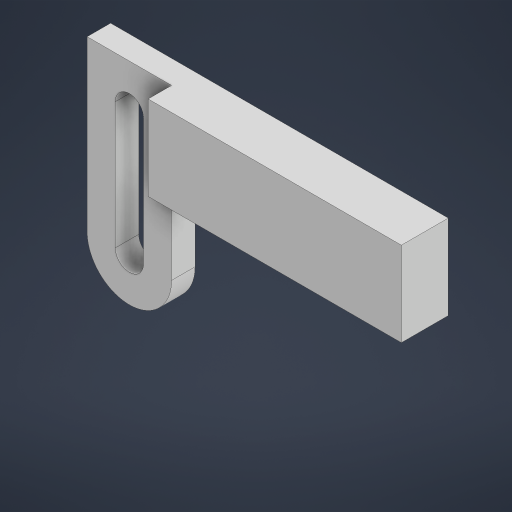
# Autodesk Inventor part: Slider
Saved by Autodesk Inventor 2024 (Build 280153000, 153)
## iProperties
Created: 2024-02-01
Part Number: Slider
Material: Generic
Document SubType Name: Modeling
Designer: calvi
Density: 1 g/cm^3
Appearance: Default
Author: calvi
Autodesk Inventor part; units mm, degrees
ref_plane "YZ Plane" through (0, 0, 0) normal (1, 0, 0) x (0, 1, 0)
ref_plane "XZ Plane" through (0, 0, 0) normal (0, 1, 0) x (-1, 0, 0)
ref_plane "XY Plane" through (0, 0, 0) normal (0, 0, 1) x (1, 0, 0)
sketch "Sketch3" plane through (0, 0, 0) normal (0, 0, 1) x (1, 0, 0)
  line L0 (0, 0) -> (22.86, 0)
  line L1 (22.86, 0) -> (22.86, 91.44)
  line L2 (22.86, 91.44) -> (0, 91.44)
  line L3 (0, 91.44) -> (0, 0)
  line L4 (22.86, 57.15) -> (91.44, 57.15)
  line L5 (91.44, 57.15) -> (91.44, 34.29)
  line L6 (91.44, 34.29) -> (22.86, 34.29)
  line L7 (22.86, 34.29) -> (22.86, 57.15)
  line L8 (11.43, 80.01) -> (11.43, 11.43) construction
  line L9 (7.62, 80.01) -> (7.62, 11.43)
  line L10 (15.24, 11.43) -> (15.24, 80.01)
  arc A0 (15.24, 80.01) -> (7.62, 80.01) centre (11.43, 80.01) ccw
  arc A1 (7.62, 11.43) -> (15.24, 11.43) centre (11.43, 11.43) ccw
  arc A2 (22.86, 80.01) -> (0, 80.01) centre (11.43, 80.01) ccw
  arc A3 (0, 11.43) -> (22.86, 11.43) centre (11.43, 11.43) ccw
  point P0 (11.43, 45.72)
  point P1 (22.86, 34.29)
  dimension "d15" = 22.86
  dimension "d16" = 91.44
  dimension "d17" = 68.58
  dimension "d18" = 22.86
  dimension "d19" = 34.29
  dimension "d22" = 68.58
  dimension "d23" = 7.62
  dimension "d24" = 11.43
  dimension "d25" = 11.43
  constraints: 24 end point, 8 point on circle, 6 tangent, 5 parallel, 5 point on line, 4 centre point, 2 coincident, 2 horizontal, 2 perpendicular, 1 midpoint, 1 vertical
  measures "d15" distance of L2.end L1.end
  measures "d16" distance of L1.end L0.end
  measures "d17" distance of L5.end L6.end
  measures "d18" distance of L4.end L5.end
  measures "d19" distance between parallel lines of L4 L2
  measures "d22" distance of L8.start L8.end
  measures "d23" diameter of A1
  measures "d24" distance from line of L2 L8.start
  measures "d25" distance from line of L3 L8.start
extrude "Extrusion3" add sketch "Sketch3" against normal blind 12.7 contours A3 L3 A2 L1 | L1 L4 L5 L6
sketch "Sketch5" plane through (0, 0, 0) normal (0, 0, 1) x (1, 0, 0)
  line L0 (0, 0) -> (22.86, 0)
  line L1 (22.86, 0) -> (22.86, 91.44)
  line L2 (22.86, 91.44) -> (0, 91.44)
  line L3 (0, 91.44) -> (0, 0)
  arc A0 (22.86, 80.01) -> (0, 80.01) centre (11.43, 80.01) ccw projected
  line L4 (22.86, 57.15) -> (22.86, 80.01) projected
  dimension "d30" = 0
  constraints: 8 end point, 2 parallel, 1 horizontal, 1 perpendicular, 1 tangent
  measures "d30" distance between parallel lines of L1 L4
extrude "Extrusion5" cut sketch "Sketch5" against normal blind 6.35 contours L3 A0 L1 L0
sketch "Sketch7" plane through (0, 0, -6.35) normal (0, 0, 1) x (1, 0, 0)
  line L0 (91.44, 57.15) -> (22.86, 57.15) projected
  line L1 (22.86, 57.15) -> (0, 57.15)
  line L2 (0, 57.15) -> (0, 91.44)
  line L3 (0, 91.44) -> (22.86, 91.44)
  line L4 (22.86, 91.44) -> (22.86, 57.15)
  line L5 (0, 11.43) -> (0, 80.01) projected
  arc A0 (22.86, 80.01) -> (0, 80.01) centre (11.43, 80.01) ccw projected
  point P0 (0, 0)
  dimension "d36" = 0
  constraints: 8 end point, 2 parallel, 1 horizontal, 1 perpendicular, 1 tangent
  measures "d36" distance between parallel lines of L5 L2
extrude "Extrusion6" cut sketch "Sketch7" against normal blind 88.9 contours L1 L2 A0 L4
sketch "Sketch8" plane through (0, 0, -6.35) normal (0, 0, 1) x (1, 0, 0)
  line L0 (22.86, 57.15) -> (0, 57.15)
  line L1 (0, 57.15) -> (0, 41.91)
  line L2 (22.86, 41.91) -> (22.86, 57.15)
  line L3 (0, 11.43) -> (0, 57.15) projected
  line L4 (15.24, 11.43) -> (15.24, 57.15) projected
  arc A0 (15.24, 45.72) -> (7.62, 45.72) centre (11.43, 45.72) ccw
  line L5 (7.62, 57.15) -> (7.62, 11.43) projected
  line L6 (0, 41.91) -> (7.62, 41.91)
  line L7 (15.24, 41.91) -> (22.86, 41.91)
  line L8 (15.24, 45.72) -> (15.24, 41.91)
  line L9 (15.24, 11.43) -> (15.24, 57.15) projected
  line L10 (7.62, 45.72) -> (7.62, 41.91)
  point P0 (0, 0)
  point P1 (11.43, 57.15)
  dimension "d40" = 0
  dimension "d42" = 7.62
  dimension "d43" = 15.24
  constraints: 14 end point, 4 point on line, 3 parallel, 3 tangent, 2 collinear, 2 point on circle, 1 centre point, 1 horizontal, 1 midpoint, 1 perpendicular
  measures "d40" distance between parallel lines of L3 L1
  measures "d42" diameter of A0
  measures "d43" distance between parallel lines of L0 L6
extrude "Extrusion7" add sketch "Sketch8" against normal blind 6.35 contours L4 A0 L5 L0
body "Solid2"
